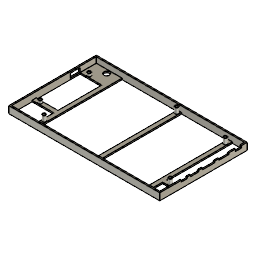
Mini PC Case V4 (Autodesk Fusion 360 design; units mm, degrees)
Autodesk Fusion 360 part; units mm, degrees
sketch "Sketch1" plane through (0, 0, 0) normal (0, 0, 1) x (1, 0, 0)
  line L0 (0, 0) -> (210, 0)
  line L1 (210, 0) -> (210, 120)
  line L2 (210, 120) -> (0, 120)
  line L3 (0, 120) -> (0, 0)
  line L4 (190, 120) -> (190, 0) construction
  line L5 (118, 120) -> (118, 0) construction
  line L6 (118, 113) -> (210, 113) construction
  line L7 (118, 24) -> (210, 24) construction
  line L8 (118, 116) -> (210, 116) construction
  circle A0 centre (118, 116) radius 1.65
  circle A1 centre (190, 113) radius 1.65
  line L9 (-2, 122) -> (-2, -2)
  line L10 (-2, -2) -> (212, -2)
  line L11 (212, -2) -> (212, 122)
  line L12 (212, 122) -> (-2, 122)
  line L13 (115, 120) -> (115, 0)
  line L14 (121, 120) -> (121, 0)
  line L15 (187, 120) -> (187, 0)
  line L16 (193, 120) -> (193, 0)
  line L17 (33.7, 120) -> (33.7, 0) construction
  line L18 (30.7, 120) -> (30.7, 0)
  line L19 (36.7, 120) -> (36.7, 0)
  line L20 (201, 120) -> (201, 0) construction
  circle A2 centre (201, 24) radius 1.65
  line L21 (118, 21) -> (210, 21)
  line L22 (118, 27) -> (210, 27)
  line L23 (33.7, 120) -> (33.7, 0) construction
  circle A3 centre (33.7, 12.5) radius 1.65
  line L24 (210, 113.8) -> (212, 113.8)
  line L25 (210, 105.5) -> (212, 105.5)
  line L26 (210, 96) -> (212, 96)
  line L27 (210, 82) -> (212, 82)
  line L28 (210, 76) -> (212, 76)
  line L29 (210, 59) -> (212, 59)
  line L30 (210, 53) -> (212, 53)
  line L31 (210, 42) -> (212, 42)
  line L32 (210, 37) -> (212, 37)
  line L33 (210, 29) -> (212, 29)
  circle A4 centre (33.7, 12.5) radius 2.5
  circle A5 centre (201, 24) radius 2.5
  circle A6 centre (190, 113) radius 2.5
  circle A7 centre (118, 116) radius 2.5
  circle A8 centre (10, 100) radius 1.65
  circle A9 centre (8.7, 32) radius 1.65
  circle A10 centre (10, 100) radius 2.5
  circle A11 centre (8.7, 32) radius 2.5
  line L34 (0, 100) -> (33.7, 100) construction
  line L35 (0, 32) -> (33.7, 32) construction
  line L36 (0, 97) -> (33.7, 97)
  line L37 (0, 103) -> (33.7, 103)
  line L38 (0, 29) -> (33.7, 29)
  line L39 (0, 35) -> (33.7, 35)
  line L40 (0, 97) -> (-2, 97)
  line L41 (-2, 83.5) -> (0, 83.5)
  circle A12 centre (20, 114.7) radius 4
  dimension "d1" = 210
  dimension "d2" = 120
  dimension "d3" = 20
  dimension "d4" = 92
  dimension "d5" = 7
  dimension "d6" = 96
  dimension "d7" = 4
  dimension "d8" = 3.3
  dimension "d9" = 3.3
  dimension "d11" = 2
  dimension "d12" = 3
  dimension "d13" = -3
  dimension "d14" = 3
  dimension "d15" = -3
  dimension "d17" = 3
  dimension "d18" = -3
  dimension "d21" = 9
  dimension "d24" = 3.3
  dimension "d25" = 3
  dimension "d26" = -3
  dimension "d29" = 3.3
  dimension "d31" = 107.5
  dimension "d32" = 176.3
  dimension "d33" = 6.2
  dimension "d34" = 14.5
  dimension "d35" = 24
  dimension "d36" = 38
  dimension "d37" = 44
  dimension "d38" = 61
  dimension "d39" = 67
  dimension "d40" = 78
  dimension "d41" = 83
  dimension "d42" = 91
  dimension "d46" = 5
  dimension "d48" = 5
  dimension "d49" = 5
  dimension "d50" = 5
  dimension "d53" = 3.3
  dimension "d54" = 20
  dimension "d55" = 10
  dimension "d56" = 3.3
  dimension "d57" = 88
  dimension "d58" = 8.7
  dimension "d59" = 5
  dimension "d60" = 5
  dimension "d61" = 3
  dimension "d62" = -3
  dimension "d63" = 3
  dimension "d64" = -3
  dimension "d65" = 23
  dimension "d66" = 36.5
  dimension "d67" = 8
  dimension "d68" = 20
  dimension "d69" = 5.3
  constraint horizontal L0
  constraint vertical L1
  constraint horizontal L2
  constraint vertical L3
  constraint coincident L0.start L3.end
  constraint coincident L2 L4.start
  constraint coincident L0 L4.end
  constraint perpendicular L0 L4
  constraint coincident L2 L5.start
  constraint coincident L0 L5.end
  constraint perpendicular L0 L5
  constraint coincident L5 L6.start
  constraint coincident L1 L6.end
  constraint perpendicular L1 L6
  constraint coincident L5 L7.start
  constraint coincident L1 L7.end
  constraint perpendicular L1 L7
  constraint coincident L5 L8.start
  constraint coincident L1 L8.end
  constraint perpendicular L1 L8
  constraint coincident L8.start A0.centre
  constraint coincident L4 A1.centre
  constraint coincident L6 A1.centre
  constraint coincident L2 L17.start
  constraint coincident L0 L17.end
  constraint perpendicular L0 L17
  constraint coincident L2 L20.start
  constraint coincident L0 L20.end
  constraint perpendicular L0 L20
  constraint coincident L20 A2.centre
  constraint coincident L7 A2.centre
  constraint perpendicular L0 L23
  constraint coincident L23 A3.centre
  constraint coincident L1 L24.start
  constraint coincident L11 L24.end
  constraint perpendicular L11 L24
  constraint coincident L1 L25.start
  constraint coincident L11 L25.end
  constraint perpendicular L11 L25
  constraint coincident L1 L26.start
  constraint coincident L11 L26.end
  constraint perpendicular L11 L26
  constraint coincident L1 L27.start
  constraint coincident L11 L27.end
  constraint perpendicular L11 L27
  constraint coincident L1 L28.start
  constraint coincident L11 L28.end
  constraint perpendicular L11 L28
  constraint coincident L1 L29.start
  constraint coincident L11 L29.end
  constraint perpendicular L11 L29
  constraint coincident L1 L30.start
  constraint coincident L11 L30.end
  constraint perpendicular L11 L30
  constraint coincident L1 L31.start
  constraint coincident L11 L31.end
  constraint perpendicular L11 L31
  constraint coincident L1 L32.start
  constraint coincident L11 L32.end
  constraint perpendicular L11 L32
  constraint coincident L1 L33.start
  constraint coincident L11 L33.end
  constraint perpendicular L11 L33
  constraint coincident L5 L21.start
  constraint coincident L5 L22.start
  constraint collinear L17 L23
  constraint concentric A3 A4
  constraint concentric A2 A5
  constraint concentric A1 A6
  constraint concentric A0 A7
  constraint concentric A8 A10
  constraint concentric A9 A11
  constraint coincident L3 L34.start
  constraint coincident L23 L34.end
  constraint perpendicular L23 L34
  constraint coincident L3 L35.start
  constraint coincident L23 L35.end
  constraint perpendicular L23 L35
  constraint coincident L3 L36.start
  constraint coincident L9 L40.end
  constraint perpendicular L9 L40
  constraint coincident L9 L41.start
  constraint coincident L3 L41.end
  constraint perpendicular L3 L41
  measures "d1" distance of L0.start L0.end
  measures "d2" distance of L0.start L2.end
  measures "d3" distance of L1 L4
  measures "d4" distance of L1 L5
  measures "d5" distance of L2 L6
  measures "d6" distance of L2 L7
  measures "d7" distance of L2 L8
  measures "d8" diameter of A0
  measures "d9" diameter of A1
  measures "d21" distance of L1 L20
  measures "d24" diameter of A2
  measures "d29" diameter of A3
  measures "d31" distance of L2 A3.centre
  measures "d32" distance of L1 L17
  measures "d33" distance of L1.end L24
  measures "d34" distance of L1.end L25
  measures "d35" distance of L1.end L26
  measures "d36" distance of L1.end L27
  measures "d37" distance of L1.end L28
  measures "d38" distance of L1.end L29
  measures "d39" distance of L1.end L30
  measures "d40" distance of L1.end L31
  measures "d41" distance of L1.end L32
  measures "d42" distance of L1.end L33
  measures "d46" diameter of A4
  measures "d48" diameter of A5
  measures "d49" diameter of A6
  measures "d50" diameter of A7
  measures "d53" diameter of A8
  measures "d54" distance of L2 A8.centre
  measures "d55" distance of L3 A8.centre
  measures "d56" diameter of A9
  measures "d57" distance of L2 A9.centre
  measures "d58" distance of L3 A9.centre
  measures "d59" diameter of A10
  measures "d60" diameter of A11
  measures "d65" distance of L2 L40
  measures "d66" distance of L2 L41
  measures "d67" diameter of A12
  measures "d68" distance of L3 A12.centre
  measures "d69" distance of L2 A12.centre
extrude "Extrude1" add sketch "Sketch1" along normal blind 2 contours L0 L1 L3 L9 L10 L11 L33 L41 | L0 L2 L18 L19 | L3 L18 L38 L39 | L0 L2 L13 L14 | L1 L2 L3 L9 L11 L12 L24 L40 | L3 L9 L40 L41 | L2 L3 L18 L37 | L3 L18 L36 L37 | L0 L15 L16 L21 | L15 L16 L21 L22 | L2 L15 L16 L22 | L1 L16 L21 L22 | L1 L11 L32 L33 | L1 L11 L24 L25 | L1 L11 L31 L32 | L1 L11 L25 L26 | L1 L11 L30 L31 | L1 L11 L26 L27 | L1 L11 L29 L30 | L1 L11 L27 L28 | L1 L11 L28 L29 | A4 | A5 | A6 | A7 | A10 | A11
extrude "Extrude2" add sketch "Sketch1" along normal blind 10 contours L0 L1 L3 L9 L10 L11 L33 L41 | L1 L2 L3 L9 L11 L12 L24 L40 | L1 L11 L31 L32 | L1 L11 L25 L26 | L1 L11 L29 L30 | L1 L11 L27 L28
extrude "Extrude3" add sketch "Sketch1" along normal blind 10 contours A4 | A5 | A6 | A7
extrude "Extrude4" add sketch "Sketch1" along normal blind 6 contours A10 | A11
extrude "Extrude5" add 4 faces at (210.6667, 86.6667, 2) (211.3333, 64.6667, 2) (211.3333, 45.6667, 2) (211.3333, 31.6667, 2) along direction (0, 0, 1) blind 6
extrude "Extrude6" add 1 faces at (210.6667, 111.0333, 2) along direction (0, 0, 1) blind 5
extrude "Extrude7" add 1 faces at (-0.6667, 92.5, 2) along direction (0, 0, 1) blind 8 and the other way blind -6
equation "d8 = HolesRadius"
equation "d9 = HolesRadius"
equation "d24 = HolesRadius"
equation "d29 = HolesRadius"
equation "HolesRadius = 3.3 mm"
equation "d46 = HolesOuterRadius"
equation "HolesOuterRadius = 5 mm"
equation "d48 = HolesOuterRadius"
equation "d49 = HolesOuterRadius"
equation "d50 = HolesOuterRadius"
equation "d53 = HolesRadius"
equation "d56 = HolesRadius"
equation "d59 = HolesOuterRadius"
equation "d60 = HolesOuterRadius"
